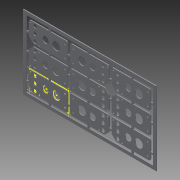
# Autodesk Inventor part: Granny Gearbox Output Plate Routing Template (9-up)
Saved by Autodesk Inventor 2015 (Build 190159000, 159)
## iProperties
Created: 2016-02-25
Part Number: Granny Gearbox Output Plate Routing Template (9-up)
Material: Generic
Document SubType Name: Modeling
Designer: sethbattis
Density: 1 g/cm^3
Appearance: Default
Author: sethbattis
Autodesk Inventor part; units mm, degrees
ref_plane "YZ Plane" through (0, 0, 0) normal (1, 0, 0) x (0, 1, 0)
ref_plane "XZ Plane" through (0, 0, 0) normal (0, 1, 0) x (-1, 0, 0)
ref_plane "XY Plane" through (0, 0, 0) normal (0, 0, 1) x (1, 0, 0)
derived "Granny Gearbox Output Plate.ipt"
sketch "New Mounting Holes" plane through (0, 0, 0) normal (0, 0, 1) x (1, 0, 0)
  circle A0 centre (74.3367, 23.3553) radius 3.175
  circle A1 centre (74.3367, -23.3553) radius 3.175
  circle A2 centre (-57.7242, 30.4609) radius 3.175
  circle A3 centre (-24.3812, -30.912) radius 3.175
  line L0 (-65.3633, -38.1) -> (-65.3633, 38.1) construction
  line L1 (87.0367, -38.1) -> (-65.3633, -38.1) construction
  line L2 (87.0367, 38.1) -> (87.0367, -38.1) construction
  line L3 (-65.3633, 38.1) -> (87.0367, 38.1) construction
  line L4 (-55.8383, 38.1) -> (-55.8383, -38.1) construction
  line L5 (-65.3633, 28.575) -> (87.0367, 28.575) construction
  line L6 (-65.3633, -28.575) -> (87.0367, -28.575) construction
  line L7 (77.5117, 38.1) -> (77.5117, -38.1) construction
  circle A4 centre (-40.7035, -0.0359) radius 31.75 construction
  circle A5 centre (40.6908, 0) radius 36.195 construction
  circle A6 centre (0, 0) radius 36.195 construction
  line L8 (-57.7242, 30.4609) -> (-55.8383, 30.4609) construction
  line L9 (-57.7242, 30.4609) -> (-57.7242, 28.575) construction
sketch "Labels" plane through (0, 0, 0) normal (0, 0, 1) x (1, 0, 0)
  circle A0 centre (-40.7035, -0.0359) radius 5.5626
  circle A1 centre (-40.7035, 25.3641) radius 5.5626
  circle A2 centre (-40.7035, -25.4359) radius 5.5626
  circle A3 centre (0, 0) radius 11.1125
  circle A4 centre (40.6908, 0) radius 14.2875
  line L0 (-5.8677, 26.2224) -> (48.5566, 26.2224) construction
  line L1 (48.5566, 26.2224) -> (48.5566, 22.1963) construction
  line L2 (48.5566, 22.1963) -> (-5.8677, 22.1963) construction
  line L3 (-5.8677, 22.1963) -> (-5.8677, 26.2224) construction
sketch "Exterior" plane through (0, 0, 0) normal (0, 0, 1) x (1, 0, 0)
  line L0 (-59.0133, 38.1) -> (80.6867, 38.1)
  line L1 (87.0367, 31.75) -> (87.0367, -31.75)
  line L2 (80.6867, -38.1) -> (-44.6678, -38.1)
  arc A0 (87.0367, 31.75) -> (80.6867, 38.1) centre (80.6867, 31.75) ccw
  arc A1 (80.6867, -38.1) -> (87.0367, -31.75) centre (80.6867, -31.75) ccw
  arc A2 (-59.0133, 38.1) -> (-65.3633, 31.75) centre (-59.0133, 31.75) ccw
  circle A3 centre (-40.7035, -0.0359) radius 31.75 construction
  line L3 (-65.3633, -17.4045) -> (-65.3633, 31.75)
  line L4 (-63.5034, -21.8946) -> (-49.1579, -36.2401)
  line L5 (-65.3633, -38.1) -> (-65.3633, 38.1) construction
  line L6 (87.0367, -38.1) -> (-65.3633, -38.1) construction
  arc A4 (-49.1579, -36.2401) -> (-44.6678, -38.1) centre (-44.6678, -31.75) ccw
  arc A5 (-65.3633, -17.4045) -> (-63.5034, -21.8946) centre (-59.0133, -17.4045) ccw
  point P0 (87.0367, 38.1)
  point P1 (-65.3633, -20.0348)
  point P2 (-47.2981, -38.1)
sketch "Sketch1" plane through (0, 0, 0) normal (0, 0, 1) x (1, 0, 0)
  circle A0 centre (-57.7242, 30.4609) radius 3.175 projected
  circle A1 centre (74.3367, 23.3553) radius 3.175 projected
  circle A2 centre (74.3367, -23.3553) radius 3.175 projected
  circle A3 centre (-24.3812, -30.912) radius 3.175 projected
  circle A4 centre (-40.7035, 25.3641) radius 7.0866
  circle A5 centre (-40.7035, -0.0359) radius 7.0866
  circle A6 centre (-40.7035, -25.4359) radius 7.0866
  circle A7 centre (0, 0) radius 12.6365
  circle A8 centre (40.6908, 0) radius 15.8115
  circle A9 centre (74.3367, 23.3553) radius 3.175
  circle A10 centre (74.3367, -23.3553) radius 3.175
  circle A11 centre (-24.3812, -30.912) radius 3.175
  circle A12 centre (-57.7242, 30.4609) radius 3.175
  circle A13 centre (-40.7035, -0.0359) radius 5.5626 projected
  circle A14 centre (-40.7035, -25.4359) radius 5.5626 projected
  circle A15 centre (-40.7035, 25.3641) radius 5.5626 projected
  circle A16 centre (0, 0) radius 11.1125 projected
  circle A17 centre (40.6908, 0) radius 14.2875 projected
  line L0 (-57.4893, 36.576) -> (12.6365, 36.576)
  line L1 (85.5127, 30.226) -> (85.5127, -5.069)
  line L2 (79.1627, -36.576) -> (18.9865, -36.576)
  line L3 (-65.3633, 38.1) -> (87.0367, 38.1) construction
  line L4 (87.0367, 38.1) -> (87.0367, -38.1) construction
  line L5 (87.0367, -38.1) -> (-65.3633, -38.1) construction
  line L6 (-63.5034, -21.8946) -> (-49.1579, -36.2401) projected
  line L7 (-65.3633, -38.1) -> (-65.3633, 38.1) construction
  line L8 (-61.9794, -21.2634) -> (-48.5267, -34.7161)
  line L9 (-63.8393, -16.7732) -> (-63.8393, -11.419)
  arc A18 (-57.4893, 36.576) -> (-63.8393, 30.226) centre (-57.4893, 30.226) ccw
  arc A19 (-63.8393, -16.7732) -> (-61.9794, -21.2634) centre (-57.4893, -16.7732) ccw
  arc A20 (-48.5267, -34.7161) -> (-44.0365, -36.576) centre (-44.0365, -30.226) ccw
  arc A21 (79.1627, -36.576) -> (85.5127, -30.226) centre (79.1627, -30.226) ccw
  arc A22 (85.5127, 30.226) -> (79.1627, 36.576) centre (79.1627, 30.226) ccw
  line L10 (18.9865, 36.576) -> (18.9865, 41.3004)
  line L11 (18.9865, 41.3004) -> (12.6365, 41.3004)
  line L12 (12.6365, 41.3004) -> (12.6365, 36.576)
  line L13 (18.9865, -36.576) -> (18.9865, -41.3004)
  line L14 (18.9865, -41.3004) -> (12.6365, -41.3004)
  line L15 (12.6365, -41.3004) -> (12.6365, -36.576)
  line L16 (85.5127, -11.419) -> (90.2371, -11.419)
  line L17 (90.2371, -11.419) -> (90.2371, -5.069)
  line L18 (90.2371, -5.069) -> (85.5127, -5.069)
  line L19 (-63.8393, -11.419) -> (-68.5637, -11.419)
  line L20 (-68.5637, -11.419) -> (-68.5637, -5.069)
  line L21 (-68.5637, -5.069) -> (-63.8393, -5.069)
  line L22 (18.9865, 36.576) -> (79.1627, 36.576)
  line L23 (85.5127, -11.419) -> (85.5127, -30.226)
  line L24 (12.6365, -36.576) -> (-44.0365, -36.576)
  line L25 (-63.8393, -5.069) -> (-63.8393, 30.226)
  dimension "d15" = 1.524
  dimension "d18" = 1.524
  dimension "d19" = 1.524
  dimension "d21" = 1.524
  dimension "d22" = 6.35
  dimension "d23" = 28.575
  dimension "d24" = 31.623
  dimension "d25" = 22.225
  dimension "d26" = 25.273
  dimension "d27" = 11.1252
  dimension "d28" = 14.1732
  dimension "d31" = 6.35
  dimension "d34" = 4.7244
  constraints: 42 end point, 18 tangent, 14 centre point, 13 parallel, 10 equal radius, 10 point on circle, 9 coincident, 6 perpendicular, 5 concentric, 5 equal length, 4 horizontal, 4 point on line, 1 collinear
  measures "d15" distance between parallel lines of L0 L3
  measures "d18" distance between parallel lines of L1 L4
  measures "d19" distance between parallel lines of L5 L2
  measures "d21" distance between parallel lines of L8 L6
  measures "d22" radius of A18
  measures "d23" diameter of A17
  measures "d24" diameter of A8
  measures "d25" diameter of A16
  measures "d26" diameter of A7
  measures "d27" diameter of A15
  measures "d28" diameter of A4
  measures "d31" distance of L11.end L10.end
  measures "d34" distance of L10.start L10.end
extrude "Extrusion1" add sketch "Sketch1" along normal blind 3.175 contours L0 L12 L11 L10 L22 A22 L1 L18 L17 L16 L23 A21 L2 L13 L14 L15 L24 A20 L8 A19 L9 L19 L20 L21 L25 A18
mirror "Mirror1" about plane through (90.2371, -11.419, 0) normal (1, 0, 0)
mirror "Mirror2" about plane through (249.0379, -5.069, 0) normal (1, 0, 0) of "Mirror1"
mirror "Mirror3" about plane through (161.4877, 41.3004, 0) normal (0, 1, 0)
mirror "Mirror4" about plane through (330.2381, 123.9012, 0) normal (0, 1, 0) of "Mirror3"
sketch "Sketch5" plane through (0, 0, 0) normal (0, 0, 1) x (1, 0, 0)
  line L0 (-73.2881, 211.2264) -> (-73.2881, 160.1326)
  line L1 (-73.2881, -46.0248) -> (-85.9881, -46.0248)
  line L2 (-85.9881, -46.0248) -> (-85.9881, 200.5697)
  line L3 (412.5631, 211.2264) -> (412.5631, 223.9264)
  line L4 (412.5631, 223.9264) -> (-85.9881, 223.9264)
  line L5 (-85.9881, 223.9264) -> (-85.9881, 200.5697)
  line L6 (-73.2881, 211.2264) -> (12.6365, 211.2264)
  line L7 (-44.0365, -36.576) -> (12.6365, -36.576) projected
  line L8 (407.8387, 153.7826) -> (407.8387, 160.1326) projected
  line L9 (12.6365, -41.3004) -> (18.9865, -41.3004) projected
  line L10 (12.6365, 206.502) -> (18.9865, 206.502)
  line L11 (18.9865, 206.502) -> (18.9865, 211.2264)
  line L12 (12.6365, 211.2264) -> (12.6365, 206.502)
  line L13 (161.4877, 206.502) -> (167.8377, 206.502)
  line L14 (167.8377, 206.502) -> (167.8377, 211.2264)
  line L15 (161.4877, 211.2264) -> (161.4877, 206.502)
  line L16 (330.2381, 206.502) -> (336.5881, 206.502)
  line L17 (336.5881, 206.502) -> (336.5881, 211.2264)
  line L18 (330.2381, 211.2264) -> (330.2381, 206.502)
  line L19 (-68.5637, 160.1326) -> (-73.2881, 160.1326)
  line L20 (-73.2881, 153.7826) -> (-68.5637, 153.7826)
  line L21 (-68.5637, 153.7826) -> (-68.5637, 160.1326)
  line L22 (-68.5637, 160.1326) -> (-68.5637, 153.7826) projected
  line L23 (-68.5637, 94.0198) -> (-73.2881, 94.0198)
  line L24 (-73.2881, 87.6698) -> (-68.5637, 87.6698)
  line L25 (-68.5637, 87.6698) -> (-68.5637, 94.0198)
  line L26 (-68.5637, -5.069) -> (-73.2881, -5.069)
  line L27 (-73.2881, -11.419) -> (-68.5637, -11.419)
  line L28 (-68.5637, -11.419) -> (-68.5637, -5.069)
  line L29 (-73.2881, -11.419) -> (-73.2881, -46.0248)
  line L30 (-73.2881, 87.6698) -> (-73.2881, -5.069)
  line L31 (-73.2881, 153.7826) -> (-73.2881, 94.0198)
  line L32 (18.9865, 211.2264) -> (161.4877, 211.2264)
  line L33 (167.8377, 211.2264) -> (330.2381, 211.2264)
  line L34 (336.5881, 211.2264) -> (412.5631, 211.2264)
  point P0 (0, 0)
  dimension "d38" = 4.7244
  dimension "d39" = 4.7244
  dimension "d42" = 12.7
  dimension "d44" = 12.7
  dimension "d51" = 4.7244
  dimension "d52" = 4.7244
  constraints: 62 end point, 14 parallel, 11 horizontal, 9 point on line, 3 perpendicular, 1 collinear, 1 vertical
  measures "d38" distance between parallel lines of L6 L16
  measures "d39" distance between parallel lines of L22 L0
  measures "d42" distance between parallel lines of L4 L34
  measures "d44" distance between parallel lines of L2 L29
  measures "d51" distance between parallel lines of L9 L1
  measures "d52" distance between parallel lines of L3 L8
extrude "Extrusion2" add sketch "Sketch5" along normal blind 3.175
sketch "Sketch7" plane through (0, 0, 0) normal (0, 0, 1) x (1, 0, 0)
  line L0 (-85.9881, -58.7248) -> (425.2631, -58.7248)
  line L1 (412.5631, -46.0248) -> (336.5881, -46.0248)
  line L2 (-85.9881, -46.0248) -> (-85.9881, -58.7248)
  line L3 (-85.9881, 223.9264) -> (-85.9881, -46.0248) projected
  line L4 (12.6365, -41.3004) -> (18.9865, -41.3004) projected
  line L5 (412.5631, 223.9264) -> (-85.9881, 223.9264) projected
  line L6 (412.5631, 223.9264) -> (425.2631, 223.9264)
  line L7 (425.2631, 223.9264) -> (425.2631, -58.7248)
  line L8 (336.5881, -41.3004) -> (330.2381, -41.3004)
  line L9 (330.2381, -41.3004) -> (330.2381, -46.0248)
  line L10 (336.5881, -46.0248) -> (336.5881, -41.3004)
  line L11 (161.4877, -41.3004) -> (167.8377, -41.3004)
  line L12 (167.8377, -41.3004) -> (167.8377, -46.0248)
  line L13 (161.4877, -46.0248) -> (161.4877, -41.3004)
  line L14 (12.6365, -41.3004) -> (18.9865, -41.3004)
  line L15 (18.9865, -41.3004) -> (18.9865, -46.0248)
  line L16 (12.6365, -46.0248) -> (12.6365, -41.3004)
  line L17 (407.8387, 160.1326) -> (412.5631, 160.1326)
  line L18 (412.5631, 153.7826) -> (407.8387, 153.7826)
  line L19 (407.8387, -5.069) -> (412.5631, -5.069)
  line L20 (412.5631, -11.419) -> (407.8387, -11.419)
  line L21 (12.6365, -46.0248) -> (-85.9881, -46.0248)
  line L22 (161.4877, -46.0248) -> (18.9865, -46.0248)
  line L23 (330.2381, -46.0248) -> (167.8377, -46.0248)
  line L24 (412.5631, -5.069) -> (412.5631, 87.6698)
  line L25 (412.5631, 94.0198) -> (412.5631, 153.7826)
  line L26 (412.5631, 160.1326) -> (412.5631, 223.9264)
  line L27 (412.5631, -46.0248) -> (412.5631, -11.419)
  line L28 (167.8377, -36.576) -> (167.8377, -41.3004) projected
  line L29 (167.8377, -41.3004) -> (161.4877, -41.3004) projected
  line L30 (18.9865, -41.3004) -> (18.9865, -36.576) projected
  line L31 (330.2381, -36.576) -> (330.2381, -41.3004) projected
  line L32 (403.1143, -11.419) -> (407.8387, -11.419) projected
  line L33 (407.8387, -5.069) -> (407.8387, -11.419)
  line L34 (407.8387, -11.419) -> (407.8387, -5.069) projected
  line L35 (403.1143, 153.7826) -> (407.8387, 153.7826) projected
  line L36 (407.8387, 160.1326) -> (407.8387, 153.7826)
  line L37 (407.8387, 153.7826) -> (407.8387, 160.1326) projected
  line L38 (412.5631, 211.2264) -> (412.5631, 223.9264) projected
  line L39 (-85.9881, -46.0248) -> (-73.2881, -46.0248) projected
  line L40 (412.5631, 94.0198) -> (407.8387, 94.0198)
  line L41 (407.8387, 94.0198) -> (407.8387, 87.6698)
  line L42 (407.8387, 87.6698) -> (412.5631, 87.6698)
  point P0 (0, 0)
  dimension "d53" = 12.7
  dimension "d54" = 12.7
  constraints: 60 end point, 16 collinear, 13 parallel, 8 horizontal, 6 perpendicular, 3 point on line
  measures "d53" distance between parallel lines of L0 L23
  measures "d54" distance between parallel lines of L27 L7
extrude "Extrusion3" add sketch "Sketch7" along normal blind 3.175 contours L2 L21 L16 L4 L15 L22 L13 L11 L12 L23 L9 L8 L10 L1 L27 L20 L33 L19 L24 L42 L41 L40 L25 L18 L36 L17 L26 L6 L7 L0
equation "\"d18\" = d15"
equation "\"d19\" = d15"
equation "\"d21\" = d15"
equation "\"d24\" = d23 + 2 * d15"
equation "\"d26\" = d25 + 2 * d15"
equation "\"d28\" = d27 + 2 * d15"
equation "\"d38\" = d34"
equation "\"d39\" = d34"
equation "\"d51\" = d34"
equation "\"d52\" = d34"
body "Solid2"
